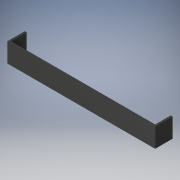
# Autodesk Inventor part: batterymount
Saved by Autodesk Inventor 2017 (Build 210142000, 142)
## iProperties
Created: 2020-02-01
Part Number: batterymount
Material: UHMW, Black
Document SubType Name: Modeling
Designer: S338674153
Density: 0.94 g/cm^3
Appearance: Smooth - Black
Author: S338674153
Autodesk Inventor part; units mm, degrees
ref_plane "YZ Plane" through (0, 0, 0) normal (1, 0, 0) x (0, 1, 0)
ref_plane "XZ Plane" through (0, 0, 0) normal (0, 1, 0) x (-1, 0, 0)
ref_plane "XY Plane" through (0, 0, 0) normal (0, 0, 1) x (1, 0, 0)
sketch "Sketch1" plane through (0, 0, 0) normal (0, 1, 0) x (-1, 0, 0)
  line L0 (0, 0) -> (215.9, 0)
  line L1 (215.9, 0) -> (215.9, -25.4)
  line L2 (215.9, -25.4) -> (0, -25.4)
  line L3 (0, -25.4) -> (0, 0)
  dimension "d0" = 215.9
  dimension "d1" = 25.4
  constraints: 8 end point, 2 parallel, 1 horizontal, 1 perpendicular
  measures "d0" distance of L1.end L2.end
  measures "d1" distance of L0.end L1.end
extrude "Extrusion1" add sketch "Sketch1" along normal blind 2.54
sketch "Sketch2" plane through (0, 2.54, 0) normal (0, 1, 0) x (1, 0, 0)
  line L0 (0, 0) -> (0, 25.4) projected
  line L1 (0, 25.4) -> (-215.9, 25.4) projected
  line L2 (0, 0) -> (-2.54, 0)
  line L3 (-2.54, 2.54) -> (-2.54, 25.4)
  line L4 (-2.54, 25.4) -> (0, 25.4)
  line L5 (0, 25.4) -> (0, 0)
  line L6 (-215.9, 25.4) -> (-215.9, 0) projected
  line L7 (0, 0) -> (-215.9, 0)
  line L8 (-215.9, 0) -> (-215.9, 2.54)
  line L9 (-213.36, 2.54) -> (-2.54, 2.54)
  line L10 (0, 2.54) -> (0, 0)
  line L11 (-215.9, 0) -> (0, 0) projected
  line L12 (-215.9, 0) -> (-213.36, 0)
  line L13 (-213.36, 2.54) -> (-213.36, 25.4)
  line L14 (-213.36, 25.4) -> (-215.9, 25.4)
  line L15 (-215.9, 25.4) -> (-215.9, 0)
  dimension "d4" = 2.54
  dimension "d5" = 2.54
  dimension "d6" = 2.54
  constraints: 24 end point, 6 parallel, 3 horizontal, 3 perpendicular, 3 point on line
  measures "d4" distance of L3.end L4.end
  measures "d5" distance of L7.end L8.end
  measures "d6" distance of L14.end L13.end
extrude "Extrusion2" add sketch "Sketch2" along normal blind 25.4 contours L2 L7 L6 L1 L13 L9 L3 L0
body "Solid1"
